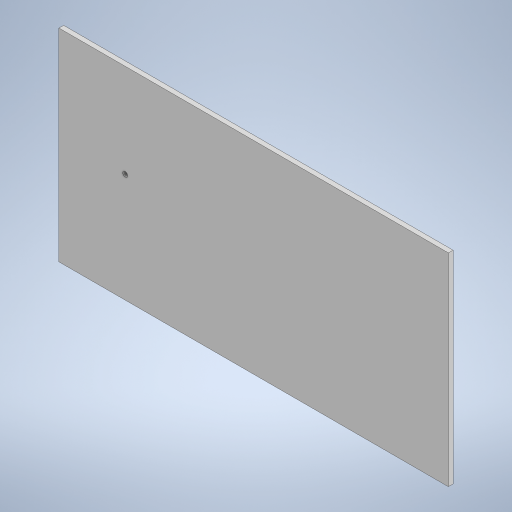
# Autodesk Inventor part: NHK_t0_11
Saved by Autodesk Inventor 2023 (Build 270158000, 158)
## iProperties
Created: 2022-04-19
Part Number: NHK_t0_11
Material: 一般
Document SubType Name: Modeling
Designer: yuta
Density: 1 g/cm^3
Appearance: 既定
Author: yuta
Autodesk Inventor part; units mm, degrees
ref_plane "YZ Plane" through (0, 0, 0) normal (1, 0, 0) x (0, 1, 0)
ref_plane "XZ Plane" through (0, 0, 0) normal (0, 1, 0) x (-1, 0, 0)
ref_plane "XY Plane" through (0, 0, 0) normal (0, 0, 1) x (1, 0, 0)
sketch "スケッチ1" plane through (0, 0, 0) normal (0, 0, 1) x (1, 0, 0)
  line L0 (0, 0) -> (85, 0)
  line L1 (85, 0) -> (85, 130)
  line L2 (85, 130) -> (0, 130)
  line L3 (0, 130) -> (0, 0)
  dimension "d0" = 85
  dimension "d1" = 130
  constraints: 8 end point, 2 parallel, 1 horizontal, 1 perpendicular
  measures "d0" distance of L2.end L1.end
  measures "d1" distance of L1.end L0.end
extrude "押し出し1" add sketch "スケッチ1" along normal blind 3
sketch "スケッチ2" plane through (0, 0, 3) normal (0, 0, 1) x (1, 0, 0)
  circle A0 centre (42.5, 70) radius 1.6
  line L0 (85, 130) -> (0, 130) projected
  line L1 (85, 0) -> (85, 130) projected
  point P0 (0, 0)
  dimension "d4" = 3.2
  dimension "d5" = 60
  dimension "d6" = 42.5
  constraints: 1 centre point
  measures "d4" diameter of A0
  measures "d5" distance from line of L0 A0.centre
  measures "d6" distance from line of L1 A0.centre
hole "穴1" at (42.5, 70, 3) direction (0, 0, -1) diameter 3.2 end through all
sketch "スケッチ3" plane through (0, 0, 3) normal (0, 0, 1) x (1, 0, 0)
  line L0 (0, 0) -> (85, 0) projected
  line L1 (85, 0) -> (250, 0)
  line L2 (250, 0) -> (250, 130)
  line L3 (250, 130) -> (85, 130)
  line L4 (85, 130) -> (85, 0)
  dimension "d14" = 165
  dimension "d15" = 130
  constraints: 8 end point, 2 parallel, 1 coincident, 1 horizontal, 1 perpendicular
  measures "d14" distance of L3.end L2.end
  measures "d15" distance of L2.end L1.end
extrude "押し出し2" add sketch "スケッチ3" against normal blind 3
